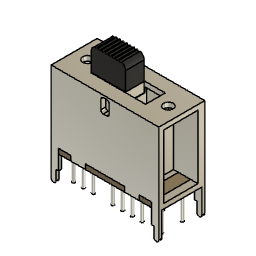
SS43D10_4P3T v7 (Autodesk Fusion 360 design; units mm, degrees)
Autodesk Fusion 360 part; units mm, degrees
note: some values were not read from the file. Set by a fixed rule: which sketch regions a step uses.
sketch "Sketch1" plane through (0, 0, 0) normal (0, 1, 0) x (1, 0, 0)
  line L0 (22, 0) -> (22, -0.5)
  line L1 (0, -0.5) -> (0, 0)
  line L2 (22, -0.5) -> (22, -3)
  line L3 (0, -3) -> (0, -0.5)
  line L4 (22, -3) -> (22, -21)
  line L5 (22, -21) -> (0, -21)
  line L6 (0, -21) -> (0, -3)
  line L7 (1, -3) -> (1, -0.5)
  line L8 (1, -0.5) -> (0, -0.5)
  line L9 (0, -0.5) -> (0, -3)
  line L10 (21, -3) -> (21, -0.5)
  line L11 (21, -0.5) -> (22, -0.5)
  line L12 (22, -0.5) -> (22, -3)
  line L13 (22, -0.5) -> (21, -0.5)
  line L14 (1, -0.5) -> (0, -0.5)
  line L15 (0, -0.5) -> (1, -0.5)
  line L16 (21, -0.5) -> (22, -0.5)
  line L17 (22, -3) -> (22, -6)
  line L18 (20.5, -6) -> (1.5, -6)
  line L19 (0, -6) -> (0, -3)
  line L20 (1.5, -6) -> (1.5, -3)
  line L21 (1.5, -3) -> (1, -3)
  line L22 (0, -3) -> (0, -6)
  line L23 (20.5, -6) -> (20.5, -3)
  line L24 (20.5, -3) -> (21, -3)
  line L25 (22, -3) -> (22, -6)
  line L26 (1, -3) -> (1.5, -3)
  line L27 (20.5, -3) -> (21, -3)
  line L28 (1, -3) -> (1.5, -3)
  line L29 (20.5, -3) -> (21, -3)
  line L30 (21, -3) -> (20.5, -3)
  line L31 (1.5, -3) -> (1, -3)
  line L32 (1.5, -6) -> (20.5, -6)
  line L33 (22, -6) -> (22, -7)
  line L34 (0, -7) -> (0, -6)
  line L35 (7, -7) -> (7, -6)
  line L36 (7, -6) -> (4, -6)
  line L37 (4, -6) -> (4, -7)
  line L38 (18, -7) -> (18, -6)
  line L39 (18, -6) -> (15, -6)
  line L40 (15, -6) -> (15, -7)
  line L41 (1.5, -7) -> (4, -7) construction
  line L42 (20.5, -7) -> (18, -7) construction
  line L43 (1.5, -6) -> (1.5, -7)
  line L44 (20.5, -6) -> (20.5, -7)
  line L45 (4, -7) -> (1.5, -7)
  line L46 (20.5, -7) -> (18, -7)
  line L47 (15, -7) -> (7, -7)
  dimension "d6" = 0.5
  dimension "d10" = 18
  dimension "d11" = 1
  dimension "d12" = 2.5
  dimension "d14" = 2.5
  dimension "d15" = 22
  dimension "d16" = 3
  dimension "d17" = 1.5
  dimension "d18" = 3
  dimension "d19" = 1.5
  dimension "d20" = 3
  dimension "d21" = 22
  dimension "d22" = 1
  dimension "d23" = 3
  dimension "d24" = 1
  dimension "d25" = 3
  dimension "d26" = 1
  dimension "d27" = 4
  dimension "d28" = 4
  constraint vertical L0
  constraint horizontal L13
  constraint vertical L1
  constraint coincident L1.end origin
  constraint horizontal L15
  constraint vertical L2
  constraint horizontal L30
  constraint vertical L3
  constraint horizontal L26
  constraint vertical L4
  constraint horizontal L5
  constraint vertical L6
  constraint vertical L7
  constraint horizontal L8
  constraint vertical L9
  constraint vertical L10
  constraint horizontal L11
  constraint vertical L12
  constraint collinear L13 L14
  constraint collinear L15 L16
  constraint horizontal L28
  constraint vertical L17
  constraint horizontal L18
  constraint vertical L19
  constraint vertical L20
  constraint horizontal L21
  constraint vertical L22
  constraint vertical L23
  constraint horizontal L24
  constraint vertical L25
  constraint collinear L26 L27
  constraint collinear L28 L29
  constraint collinear L30 L31
  constraint horizontal L32
  constraint vertical L33
  constraint horizontal L46
  constraint vertical L34
  constraint vertical L35
  constraint horizontal L36
  constraint vertical L37
  constraint vertical L38
  constraint horizontal L39
  constraint vertical L40
  constraint perpendicular L34 L41
  constraint perpendicular L4 L42
  constraint collinear L45 L46
  constraint collinear L46 L47
  measures "d6" distance of L1.end L1.start
  measures "d10" distance of L3.start L5.end
  measures "d11" distance of L3.start L7.start
  measures "d12" distance of L3.start L1.start
  measures "d14" distance of L2.end L0.end
  measures "d15" distance of L3.start L2.end
  measures "d16" distance of L3.start L19.start
  measures "d17" distance of L19.start L18.end
  measures "d18" distance of L19.start L3.start
  measures "d19" distance of L17.end L18.start
  measures "d20" distance of L17.end L2.end
  measures "d21" distance of L19.start L17.end
  measures "d22" distance of L19.start L34.start
  measures "d23" distance of L37.end L35.start
  measures "d24" distance of L37.end L36.end
  measures "d25" distance of L40.end L38.start
  measures "d26" distance of L40.end L39.end
  measures "d27" distance of L34.start L37.end
  measures "d28" distance of L33.end L38.start
extrude "Extrude1" add sketch "Sketch1" along normal blind 9.4 contours L2 L3 L4 L5 L6 L7 L8 L9 L10 L11 L12 L13 L14 L15 L16 L17 L18 L19 L20 L21 L22 L23 L24 L25 L26 L27 L28 L29 L30 L31 L32 L33 L34 L35 L36 L37 L38 L39 L40 L43 L44 L45 L46 L47 makes body 1
extrude "Extrude2" add sketch "Sketch1" along normal blind 9.4 separate body contours L18 L32 L38 L44 L46 | L18 L32 L35 L40 L47 | L18 L32 L37 L43 L45 makes body 2 at (3.1667, 3.1333, 6) makes body 3 at (9.6667, 6.2667, 6) makes body 4 at (19.6667, 3.1333, 7)
sketch "Sketch2" plane through (22, 0, 0) normal (1, 0, 0) x (0, 1, 0)
  line L0 (0, 21) -> (0, 0.5)
  line L1 (0, 0.5) -> (9.4, 0.5)
  line L2 (9.4, 0.5) -> (9.4, 21)
  line L3 (9.4, 21) -> (0, 21)
  line L4 (0, 6) -> (9.4, 6) construction
  line L5 (0, 0.5) -> (0.6, 0.5)
  line L6 (0.6, 0.5) -> (0.6, 6)
  line L7 (0.6, 6) -> (0, 6)
  line L8 (0, 6) -> (0, 0.5)
  line L9 (9.4, 0.5) -> (8.8, 0.5)
  line L10 (8.8, 0.5) -> (8.8, 6)
  line L11 (8.8, 6) -> (9.4, 6)
  line L12 (9.4, 6) -> (9.4, 0.5)
  line L13 (0.6, 6) -> (8.8, 6)
  dimension "d33" = 0.6
  dimension "d34" = 5.5
  dimension "d35" = 0.6
  dimension "d36" = 5.5
  constraint coincident L0 L4.start
  constraint coincident L2 L4.end
  constraint perpendicular L2 L4
  constraint horizontal L5
  constraint vertical L6
  constraint horizontal L7
  constraint vertical L8
  constraint coincident L0.end L1.start
  constraint horizontal L9
  constraint vertical L10
  constraint horizontal L11
  constraint vertical L12
  constraint coincident L1.end L2.start
  measures "d33" distance of L0.end L5.end
  measures "d34" distance of L0.end L4.start
  measures "d35" distance of L1.end L9.end
  measures "d36" distance of L1.end L4.end
extrude "Extrude3" cut sketch "Sketch2" against normal blind 22 contours L1 L6 L10 L13 bodies 1
fillet "Fillet1" radius 0.5 8 edges at (22, 9.1, 0.5) (21, 9.1, 0.5) (22, 0.3, 0.5) (21, 0.3, 0.5) (1, 0.3, 0.5) (0, 0.3, 0.5) (1, 9.1, 0.5) (0, 9.1, 0.5) on bodies 1
sketch "Sketch3" plane through (0, 0, 21) normal (0, 0, 1) x (-1, 0, 0)
  line L0 (0, 0) -> (-22, 0)
  line L1 (-22, 0) -> (-22, -9.4)
  line L2 (-22, -9.4) -> (0, -9.4)
  line L3 (0, -9.4) -> (0, 0)
  line L4 (2, -4.7) -> (-26, -4.7) construction
  line L5 (-11, -13) -> (-11, 2) construction
  line L6 (-2.75, -13) -> (-2.75, 2) construction
  line L7 (-19.25, -13) -> (-19.25, 2) construction
  circle A0 centre (-19.25, -4.7) radius 1
  circle A1 centre (-2.75, -4.7) radius 1
  line L8 (-16.6, -2.7) -> (-5.4, -2.7)
  line L9 (-5.4, -2.7) -> (-5.4, -6.7)
  line L10 (-5.4, -6.7) -> (-16.6, -6.7)
  line L11 (-16.6, -6.7) -> (-16.6, -2.7)
  line L12 (-16.6, -2.7) -> (-5.4, -6.7) construction
  line L13 (-5.4, -2.7) -> (-16.6, -6.7) construction
  line L14 (-5.4, -6.6) -> (-12.4, -6.6)
  line L15 (-12.4, -6.6) -> (-12.4, -2.8)
  line L16 (-12.4, -2.8) -> (-5.4, -2.8)
  line L17 (-5.4, -2.8) -> (-5.4, -6.6)
  line L18 (-5.4, -4.7) -> (-5.4, -6.6) construction
  point P0 (-11, -4.7)
  dimension "d41" = 4.7
  dimension "d42" = 11
  dimension "d45" = 8.25
  dimension "d46" = -8.25
  dimension "d47" = 2
  dimension "d48" = 2
  dimension "d49" = 11.2
  dimension "d50" = 4
  dimension "d51" = 7
  dimension "d52" = 3.8
  dimension "d53" = 1.9
  constraint parallel L2 L4
  constraint vertical L5
  constraint coincident L7 A0.centre
  constraint coincident L4 A0.centre
  constraint coincident L4 A1.centre
  constraint coincident L6 A1.centre
  constraint horizontal L8
  constraint perpendicular L8 L9
  constraint parallel L8 L10
  constraint parallel L9 L11
  constraint coincident L12 P0
  constraint coincident L13 P0
  constraint coincident L4 P0
  constraint coincident L5 P0
  constraint horizontal L14
  constraint vertical L15
  constraint horizontal L16
  constraint vertical L17
  constraint midpoint L9 L18.start
  constraint coincident L9 L14.start
  measures "d41" distance of L0 L4
  measures "d42" distance of L3 L5
  measures "d47" diameter of A0
  measures "d48" diameter of A1
  measures "d49" distance of L9.end L10.end
  measures "d50" distance of L8.end L9.end
  measures "d51" distance of L14.start L14.end
  measures "d52" distance of L14.start L16.end
  measures "d53" distance of L18.start L14.start
extrude "Extrude4" cut sketch "Sketch3" against normal blind 2 contours A0 | A1 bodies 1
extrude "Extrude5" cut sketch "Sketch3" against normal blind 2 contours L8 L9 L10 L11 L14 L15 L16 bodies 1
extrude "Extrude6" add sketch "Sketch3" along normal blind 5 separate body contours L9 L14 L15 L16 L17 makes body 5
fillet "Fillet2" radius 1.2 2 edges at (12.4, 4.7, 26) (5.4, 4.7, 26) on bodies 5
sketch "Sketch4" plane through (0, 2.8, 0) normal (0, -1, 0) x (1, 0, 0)
  arc A0 (6.6, 26) -> (5.4, 24.8) centre (6.6, 24.8) ccw
  line L0 (5.4, 24.8) -> (5.4, 21)
  line L1 (5.4, 21) -> (12.4, 21)
  line L2 (12.4, 21) -> (12.4, 24.8)
  arc A1 (12.4, 24.8) -> (11.2, 26) centre (11.2, 24.8) ccw
  line L3 (11.2, 26) -> (6.6, 26)
  circle A2 centre (6.3535, 26) radius 0.25
  circle A3 centre (7.0678, 26) radius 0.25
  circle A4 centre (7.7821, 26) radius 0.25
  circle A5 centre (8.4963, 26) radius 0.25
  circle A6 centre (9.2106, 26) radius 0.25
  circle A7 centre (9.9249, 26) radius 0.25
  circle A8 centre (10.6392, 26) radius 0.25
  circle A9 centre (11.3535, 26) radius 0.25
  dimension "d62" = 0.5
  dimension "d71" = 5
  dimension "d72" = 0
  constraint coincident L3 A2.centre
  measures "d62" diameter of A2
extrude "Extrude7" cut sketch "Sketch4" against normal blind 3.8 contours A0 L3 A2 | L3 A3 | L3 A4 | A1 L3 A9 | L3 A5 | L3 A8 | L3 A6 | L3 A7 picked at (6.3669, 25.899) picked at (7.1511, 25.8557) picked at (7.8422, 25.9309) picked at (11.4086, 25.9079) picked at (8.4334, 25.8587) picked at (10.5762, 25.8587) picked at (9.1699, 25.9154) picked at (9.8619, 25.8587) bodies 5
sketch "Sketch5" plane through (0, 0, 0) normal (0, -1, 0) x (1, 0, 0)
  arc A0 (0, 1) -> (1, 1) centre (0.5, 1) ccw
  line L0 (1, 1) -> (1, 3)
  line L1 (1, 3) -> (1.5, 3)
  line L2 (1.5, 3) -> (1.5, 6)
  line L3 (1.5, 6) -> (1.5, 7)
  line L4 (1.5, 7) -> (4, 7)
  line L5 (4, 7) -> (4, 6)
  line L6 (4, 6) -> (7, 6)
  line L7 (7, 6) -> (7, 7)
  line L8 (7, 7) -> (15, 7)
  line L9 (15, 7) -> (15, 6)
  line L10 (15, 6) -> (18, 6)
  line L11 (18, 6) -> (18, 7)
  line L12 (18, 7) -> (20.5, 7)
  line L13 (20.5, 7) -> (20.5, 6)
  line L14 (20.5, 6) -> (20.5, 3)
  line L15 (20.5, 3) -> (21, 3)
  line L16 (21, 3) -> (21, 1)
  arc A1 (21, 1) -> (22, 1) centre (21.5, 1) ccw
  line L17 (22, 1) -> (22, 21)
  line L18 (22, 21) -> (0, 21)
  line L19 (0, 21) -> (0, 1)
  line L20 (-2, 21) -> (-2, 19.1) construction
  line L21 (-2, 19.1) -> (28, 19.1) construction
  line L22 (11, 30) -> (11, -3) construction
  line L23 (11.85, 17.65) -> (10.15, 17.65)
  line L24 (10.15, 17.65) -> (10.15, 20.55)
  line L25 (10.15, 20.55) -> (11.85, 20.55)
  line L26 (11.85, 20.55) -> (11.85, 17.65)
  line L27 (11.85, 17.65) -> (10.15, 20.55) construction
  line L28 (10.15, 17.65) -> (11.85, 20.55) construction
  point P0 (11, 19.1)
  dimension "d75" = 1.9
  dimension "d77" = 1.7
  dimension "d78" = 2.9
  constraint perpendicular L18 L20
  constraint perpendicular L19 L21
  constraint perpendicular L21 L22
  constraint horizontal L23
  constraint perpendicular L23 L24
  constraint parallel L23 L25
  constraint parallel L24 L26
  constraint coincident L27 P0
  constraint coincident L28 P0
  constraint coincident L22 P0
  constraint coincident L21 P0
  measures "d75" distance of L20.start L20.end
  measures "d77" distance of L24.end L25.end
  measures "d78" distance of L23.end L24.end
extrude "Extrude8" cut sketch "Sketch5" against normal blind 1 contours L23 L24 L25 L26 bodies 1
sketch "Sketch6" plane through (0, 9.4, 0) normal (0, 1, 0) x (-1, 0, 0)
  arc A0 (-1, 1) -> (0, 1) centre (-0.5, 1) ccw
  line L0 (0, 1) -> (0, 21)
  line L1 (0, 21) -> (-22, 21)
  line L2 (-22, 21) -> (-22, 1)
  arc A1 (-22, 1) -> (-21, 1) centre (-21.5, 1) ccw
  line L3 (-21, 1) -> (-21, 3)
  line L4 (-21, 3) -> (-20.5, 3)
  line L5 (-20.5, 3) -> (-20.5, 6)
  line L6 (-20.5, 6) -> (-20.5, 7)
  line L7 (-20.5, 7) -> (-18, 7)
  line L8 (-18, 7) -> (-18, 6)
  line L9 (-18, 6) -> (-15, 6)
  line L10 (-15, 6) -> (-15, 7)
  line L11 (-15, 7) -> (-7, 7)
  line L12 (-7, 7) -> (-7, 6)
  line L13 (-7, 6) -> (-4, 6)
  line L14 (-4, 6) -> (-4, 7)
  line L15 (-4, 7) -> (-1.5, 7)
  line L16 (-1.5, 7) -> (-1.5, 6)
  line L17 (-1.5, 6) -> (-1.5, 3)
  line L18 (-1.5, 3) -> (-1, 3)
  line L19 (-1, 3) -> (-1, 1)
  line L20 (2, 19) -> (-25, 19) construction
  line L21 (-11, 30) -> (-11, -3) construction
  line L22 (-13, 30) -> (-13, -3) construction
  line L23 (-9, 30) -> (-9, -3) construction
  line L24 (-12.15, 17.55) -> (-13.85, 17.55)
  line L25 (-13.85, 17.55) -> (-13.85, 20.45)
  line L26 (-13.85, 20.45) -> (-12.15, 20.45)
  line L27 (-12.15, 20.45) -> (-12.15, 17.55)
  line L28 (-12.15, 17.55) -> (-13.85, 20.45) construction
  line L29 (-13.85, 17.55) -> (-12.15, 20.45) construction
  line L30 (-8.15, 17.55) -> (-9.85, 17.55)
  line L31 (-9.85, 17.55) -> (-9.85, 20.45)
  line L32 (-9.85, 20.45) -> (-8.15, 20.45)
  line L33 (-8.15, 20.45) -> (-8.15, 17.55)
  line L34 (-8.15, 17.55) -> (-9.85, 20.45) construction
  line L35 (-9.85, 17.55) -> (-8.15, 20.45) construction
  point P0 (-13, 19)
  point P1 (-9, 19)
  dimension "d81" = 2
  dimension "d82" = -2
  dimension "d83" = 1.7
  dimension "d84" = 2.9
  dimension "d85" = 1.7
  dimension "d86" = 2.9
  constraint perpendicular L2 L20
  constraint perpendicular L11 L21
  constraint horizontal L24
  constraint perpendicular L24 L25
  constraint parallel L24 L26
  constraint parallel L25 L27
  constraint coincident L28 P0
  constraint coincident L29 P0
  constraint coincident L22 P0
  constraint coincident L20 P0
  constraint horizontal L30
  constraint perpendicular L30 L31
  constraint parallel L30 L32
  constraint parallel L31 L33
  constraint coincident L34 P1
  constraint coincident L35 P1
  constraint coincident L23 P1
  constraint coincident L20 P1
  measures "d83" distance of L25.end L26.end
  measures "d84" distance of L24.end L25.end
  measures "d85" distance of L31.end L32.end
  measures "d86" distance of L30.end L31.end
extrude "Extrude9" cut sketch "Sketch6" against normal blind 2 contours L24 L25 L26 L27 | L30 L31 L32 L33 bodies 1
fillet "Fillet3" radius 0.85 8 edges at (13.85, 8.4, 17.55) (12.15, 8.4, 17.55) (8.15, 8.4, 17.55) (9.85, 8.4, 17.55) (13.85, 8.4, 20.45) (9.85, 8.4, 20.45) (12.15, 8.4, 20.45) (8.15, 8.4, 20.45) on bodies 1
fillet "Fillet4" radius 0.5 4 edges at (10.15, 0.5, 20.55) (11.85, 0.5, 20.55) (10.15, 0.5, 17.65) (11.85, 0.5, 17.65) on bodies 1
sketch "Sketch7" plane through (0, 0, 6) normal (0, 0, -1) x (1, 0, 0)
  line L0 (7, -9.4) -> (7, 0)
  line L1 (7, 0) -> (4, 0)
  line L2 (4, 0) -> (4, -9.4)
  line L3 (4, -9.4) -> (7, -9.4)
  line L4 (11, 2) -> (11, -13) construction
  line L5 (-3.5864, -4.7) -> (26, -4.7) construction
  line L6 (0, 0) -> (22, 0) construction
  line L7 (20, -2.6) -> (2, -2.6) construction
  line L8 (2, -2.6) -> (2, -6.8) construction
  line L9 (2, -6.8) -> (20, -6.8) construction
  line L10 (20, -6.8) -> (20, -2.6) construction
  line L11 (20, -2.6) -> (2, -6.8) construction
  line L12 (2, -2.6) -> (20, -6.8) construction
  circle A0 centre (2, -2.6) radius 0.3
  circle A1 centre (4, -2.6) radius 0.3
  circle A2 centre (6, -2.6) radius 0.3
  circle A3 centre (10, -2.6) radius 0.3
  circle A4 centre (12, -2.6) radius 0.3
  circle A5 centre (14, -2.6) radius 0.3
  circle A6 centre (16, -2.6) radius 0.3
  circle A7 centre (20, -2.6) radius 0.3
  circle A8 centre (2, -6.8) radius 0.3
  circle A9 centre (4, -6.8) radius 0.3
  circle A10 centre (6, -6.8) radius 0.3
  circle A11 centre (10, -6.8) radius 0.3
  circle A12 centre (12, -6.8) radius 0.3
  circle A13 centre (14, -6.8) radius 0.3
  circle A14 centre (16, -6.8) radius 0.3
  circle A15 centre (20, -6.8) radius 0.3
  point P0 (11, -4.7)
  dimension "d93" = 4.7
  dimension "d94" = 18
  dimension "d95" = 4.2
  dimension "d96" = 0.6
  dimension "d99" = 18
  dimension "d100" = -4.2
  constraint parallel L2 L4
  constraint horizontal L5
  constraint horizontal L7
  constraint perpendicular L7 L8
  constraint parallel L7 L9
  constraint parallel L8 L10
  constraint coincident L11 P0
  constraint coincident L12 P0
  constraint coincident L5 P0
  constraint coincident L4 P0
  constraint coincident L7.end L8.start
  measures "d93" distance of L5 L6
  measures "d94" distance of L8.end L9.end
  measures "d95" distance of L7.end L8.end
  measures "d96" diameter of A0
extrude "Extrude10" add sketch "Sketch7" along normal blind 6 separate body contours A0 | A2 | A3 | A4 | A5 | A6 | A7 | A8 | A10 | A11 | A12 | A13 | A14 | A15 makes body 6 at (15.7365, 6.6565, 2) makes body 7 at (12.256, 6.6436, 2) makes body 8 at (6.1985, 6.5751, 2) makes body 9 at (2.2996, 2.615, 2) makes body 10 at (10.2996, 2.615, 2) makes body 11 at (14.2996, 2.615, 2) makes body 12 at (20.1751, 2.3564, 2) makes body 13 at (16.2764, 2.4835, 2) makes body 14 at (12.2996, 2.615, 2) makes body 15 at (6.2996, 2.615, 2) makes body 16 at (2.1985, 6.5751, 2) makes body 17 at (10.256, 6.6436, 2) makes body 18 at (14.256, 6.6436, 2) makes body 19 at (20.1751, 6.5564, 2)
extrude "Extrude11" add sketch "Sketch7" along normal blind 6 separate body contours L2 A9 | L2 A9 | L2 A1 | L2 A1 makes body 20 at (4.2985, 2.5701, 2) makes body 21 at (4.2095, 6.5852, 4)
sketch "Sketch8" plane through (22, 0, 0) normal (1, 0, 0) x (0, 1, 0)
  line L0 (0, 1) -> (0.6, 1)
  line L1 (0.6, 1) -> (0.6, 6)
  line L2 (0.6, 6) -> (8.8, 6)
  line L3 (8.8, 6) -> (8.8, 1)
  line L4 (8.8, 1) -> (9.4, 1)
  line L5 (9.4, 1) -> (9.4, 21)
  line L6 (9.4, 21) -> (0, 21)
  line L7 (0, 21) -> (0, 1)
  line L8 (1, 20) -> (8, 20)
  line L9 (8, 20) -> (8, 7)
  line L10 (8, 7) -> (1, 7)
  line L11 (1, 7) -> (1, 20)
  constraint horizontal L8
  constraint vertical L9
  constraint horizontal L10
  constraint vertical L11
extrude "Extrude12" cut sketch "Sketch8" against normal blind 5 contours L8 L9 L10 L11 bodies 1
sketch "Sketch9" plane through (0, 0, 0) normal (-1, 0, 0) x (0, -1, 0)
  line L0 (-9.4, 1) -> (-8.8, 1)
  line L1 (-8.8, 1) -> (-8.8, 6)
  line L2 (-8.8, 6) -> (-0.6, 6)
  line L3 (-0.6, 6) -> (-0.6, 1)
  line L4 (-0.6, 1) -> (0, 1)
  line L5 (0, 1) -> (0, 21)
  line L6 (0, 21) -> (-9.4, 21)
  line L7 (-9.4, 21) -> (-9.4, 1)
  line L8 (-8, 20) -> (-1, 20)
  line L9 (-1, 20) -> (-1, 7)
  line L10 (-1, 7) -> (-8, 7)
  line L11 (-8, 7) -> (-8, 20)
  constraint horizontal L8
  constraint vertical L9
  constraint horizontal L10
  constraint vertical L11
extrude "Extrude13" cut sketch "Sketch9" against normal blind 5 contours L8 L9 L10 L11 bodies 1
sketch "Sketch10" plane through (17, 0, 0) normal (1, 0, 0) x (0, 1, 0)
  line L0 (1, 7) -> (8, 7)
  line L1 (8, 7) -> (8, 20)
  line L2 (8, 20) -> (1, 20)
  line L3 (1, 20) -> (1, 7)
  line L4 (2, 20) -> (7, 20)
  line L5 (7, 20) -> (7, 16)
  line L6 (7, 16) -> (2, 16)
  line L7 (2, 16) -> (2, 20)
  constraint horizontal L4
  constraint vertical L5
  constraint horizontal L6
  constraint vertical L7
  constraint coincident L2 L4.start
extrude "Extrude14" cut sketch "Sketch10" against normal blind 4.5 contours L2 L4 L5 L6 L7 bodies 1
sketch "Sketch11" plane through (5, 0, 0) normal (-1, 0, 0) x (0, -1, 0)
  line L0 (-8, 7) -> (-1, 7)
  line L1 (-1, 7) -> (-1, 20)
  line L2 (-1, 20) -> (-8, 20)
  line L3 (-8, 20) -> (-8, 7)
  line L4 (-7, 20) -> (-2, 20)
  line L5 (-2, 20) -> (-2, 15)
  line L6 (-2, 15) -> (-7, 15)
  line L7 (-7, 15) -> (-7, 20)
  constraint horizontal L4
  constraint vertical L5
  constraint horizontal L6
  constraint vertical L7
  constraint coincident L2 L4.start
extrude "Extrude15" cut sketch "Sketch11" against normal blind 0.3 contours L2 L4 L5 L6 L7 bodies 1
